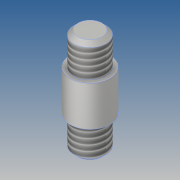
# Autodesk Inventor part: tige_serrage_main
Saved by Autodesk Inventor 2019 (Build 230136000, 136)
## iProperties
Created: 2019-04-06
Part Number: tige_serrage_main
Material: Aluminium 6061
Document SubType Name: Modeling
Designer: Theo
Density: 2.7 g/cm^3
Appearance: Aluminium - Plat
Mass: 0.52873 g
Surface Area: 2.10329 cm^2
Volume: 0.195826 cm^3
Author: Theo
Autodesk Inventor part; units mm, degrees
ref_plane "YZ Plane" through (0, 0, 0) normal (1, 0, 0) x (0, 1, 0)
ref_plane "XZ Plane" through (0, 0, 0) normal (0, 1, 0) x (-1, 0, 0)
ref_plane "XY Plane" through (0, 0, 0) normal (0, 0, 1) x (1, 0, 0)
sketch "Esquisse1" plane through (0, 0, 0) normal (0, 1, 0) x (-1, 0, 0)
  circle A0 centre (0, 0) radius 2.5
  dimension "d0" = 5
  constraints: 1 centre point, 1 coincident
  measures "d0" diameter of A0
extrude "Extrusion1" add sketch "Esquisse1" along normal mid plane 5
sketch "Esquisse2" plane through (0, -2.5, 0) normal (0, -1, 0) x (1, 0, 0)
  circle A0 centre (0, 0) radius 2
  dimension "d3" = 4
  constraints: 1 centre point, 1 coincident
  measures "d3" diameter of A0
extrude "Extrusion2" add sketch "Esquisse2" along normal blind 4
thread "Filetage1" size "M4x0.7" class "6g" standard "ISO Metric profile" full length
chamfer "Chanfrein1" distance 0.5 angle 45 1 edges at (-2, -6.5, 0)
mirror "Symétrie1" about plane through (0, 0, 0) normal (0, 1, 0) of "Extrusion2", "Chanfrein1"
